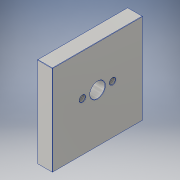
# Autodesk Inventor part: Fixture-Center
Saved by Autodesk Inventor 2016 (Build 200138000, 138)
## iProperties
Created: 2015-05-18
Part Number: Fixture-Center
Material: Generic
Document SubType Name: Modeling
Designer: jonathan
Density: 1 g/cm^3
Appearance: Aluminum - Flat
Mass: 71.5279 g
Surface Area: 160.435 cm^2
Volume: 71.5279 cm^3
Author: jonathan
Autodesk Inventor part; units mm, degrees
ref_plane "YZ Plane" through (0, 0, 0) normal (1, 0, 0) x (0, 1, 0)
ref_plane "XZ Plane" through (0, 0, 0) normal (0, 1, 0) x (-1, 0, 0)
ref_plane "XY Plane" through (0, 0, 0) normal (0, 0, 1) x (1, 0, 0)
sketch "Sketch1" plane through (0, 0, 0) normal (0, 1, 0) x (-1, 0, 0)
  line L0 (0, 0) -> (12.7, 0)
  line L1 (12.7, 0) -> (12.7, -76.2)
  line L2 (12.7, -76.2) -> (0, -76.2)
  line L3 (0, -76.2) -> (0, 0)
  dimension "d0" = 12.7
  dimension "d1" = 76.2
  constraints: 8 end point, 2 parallel, 1 horizontal, 1 perpendicular
  measures "d0" distance of L1.end L2.end
  measures "d1" distance of L0.end L1.end
extrude "Extrusion1" add sketch "Sketch1" along normal blind 76.2
sketch "Sketch2" plane through (0, 0, 0) normal (0, -1, 0) x (1, 0, 0)
  circle A0 centre (-6.35, -25.4) radius 1.27
  circle A1 centre (-6.35, -50.8) radius 1.27
  line L0 (0, 0) -> (-12.7, 0) projected
  line L1 (-12.7, -76.2) -> (0, -76.2) projected
  dimension "d4" = 2.54
  dimension "d5" = 2.54
  dimension "d6" = 25.4
  dimension "d8" = 25.4
  dimension "d9" = 6.35
  constraints: 2 centre point, 1 vertical alignment
  measures "d4" diameter of A0
  measures "d5" diameter of A1
  measures "d6" distance of A1.centre A0.centre
  measures "d8" distance from line of L1 A1.centre
  measures "d9" horizontal distance of L1.start A1.centre
extrude "Extrusion2" cut sketch "Sketch2" against normal blind 6.35
sketch "Sketch3" plane through (0, 0, 0) normal (1, 0, 0) x (0, 0, -1)
  circle A0 centre (38.1, 41.275) radius 6.35
  circle A1 centre (25.4, 41.275) radius 2.54
  line L0 (0, 0) -> (0, 76.2) projected
  circle A2 centre (50.8, 41.275) radius 2.54
  line L1 (76.2, 0) -> (0, 0) projected
  dimension "d12" = 12.7
  dimension "d13" = 5.08
  dimension "d15" = 38.1
  dimension "d16" = 25.4
  dimension "d19" = 360
  dimension "d21" = 41.275
  constraints: 3 centre point, 1 horizontal alignment, 5 other
  measures "d12" diameter of A0
  measures "d13" diameter of A1
  measures "d15" distance from line of A0.centre L0
  measures "d16" distance from line of L0 A1.centre
  measures "d21" distance from line of L1 A0.centre
extrude "Extrusion3" cut sketch "Sketch3" against normal up to next
thread "Thread1" size "12-24 UNC" class "2B" standard "ANSI Unified Screw Threads" full length
thread "Thread2" size "12-24 UNC" class "2B" standard "ANSI Unified Screw Threads" full length
chamfer "Chamfer1" distance 0.254 angle 45 18 edges at (0, 41.275, -31.75) (0, 41.275, -22.86) (0, 41.275, -48.26) (-12.7, 41.275, -48.26) (-12.7, 41.275, -31.75) (-12.7, 41.275, -22.86) (0, 76.2, -38.1) (-6.35, 76.2, 0) (-12.7, 76.2, -38.1) (0, 38.1, 0) (-12.7, 38.1, 0) (0, 38.1, -76.2) (0, 0, -38.1) (-6.35, 0, 0) (-12.7, 38.1, -76.2) (-12.7, 0, -38.1) (-6.35, 76.2, -76.2) (-6.35, 0, -76.2)
body "Solid1"
